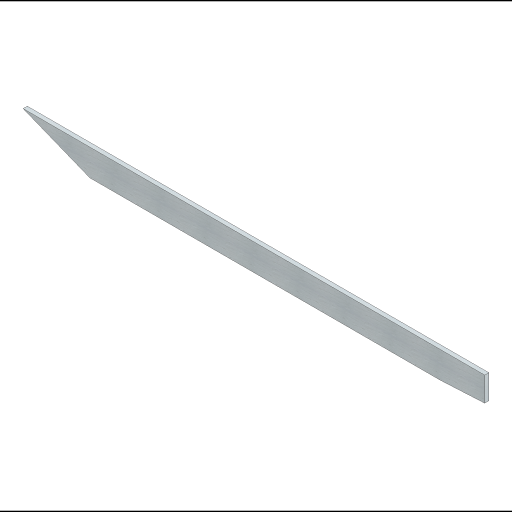
# Autodesk Inventor part: Antitorque span
Saved by Autodesk Inventor 2023 (Build 270158000, 158)
## iProperties
Created: 2023-01-26
Part Number: Antitorque span
Material: Wood (Oak)
Document SubType Name: Modeling
Designer: kamer
Density: 0.76 g/cm^3
Appearance: Wood - Painted White
Author: kamer
Autodesk Inventor part; units mm, degrees
ref_plane "YZ Plane" through (0, 0, 0) normal (1, 0, 0) x (0, 1, 0)
ref_plane "XZ Plane" through (0, 0, 0) normal (0, 1, 0) x (-1, 0, 0)
ref_plane "XY Plane" through (0, 0, 0) normal (0, 0, 1) x (1, 0, 0)
sketch "Sketch1" plane through (0, 0, 0) normal (0, 0, 1) x (1, 0, 0)
  line L0 (0, 0) -> (1320.8, 0)
  line L1 (1320.8, 0) -> (1320.8, 76.2)
  line L2 (1320.8, 76.2) -> (0, 76.2)
  line L3 (0, 76.2) -> (0, 0)
  line L4 (1193.8, 0) -> (1320.8, 6.6558)
  line L5 (0, 76.2) -> (191.0937, 0)
  dimension "d0" = 76.2
  dimension "d1" = 1320.8
  dimension "d2" = 3
  dimension "d3" = 127
  dimension "d5" = 21.74
  constraints: 12 end point, 3 point on line, 2 parallel, 1 horizontal, 1 perpendicular
  measures "d0" distance of L0.end L1.end
  measures "d1" distance of L1.end L2.end
  measures "d2" angle of L0 L4
  measures "d3" distance from line of L1 L4.start
  measures "d5" angle of L0 L5
extrude "Extrusion1" add sketch "Sketch1" along normal blind 11.938 contours L5 L2 L1 L4 L0
body "Solid1"
